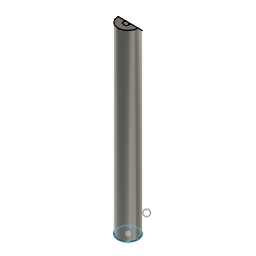
solarpanel (Autodesk Fusion 360 archive; units mm, degrees)
design "Stepper_Motor_Pole_Solar_Panel"
part number: 2025-08-02-13-12-08-452
Autodesk Fusion 360 part; units mm, degrees
sketch "Skizze1" plane through (0, 0, 0) normal (0, 0, 1) x (1, 0, 0)
  point P0 (-5.2, 16.4)
sketch "Skizze2" plane through (0, 0, 0) normal (0, 0, 1) x (1, 0, 0)
  circle A0 centre (0, 0) radius 6
extrude "Extrusion2" add sketch "Skizze2" along normal blind 110
sketch "Skizze3" plane through (0, 0, 0) normal (0, 0, 1) x (1, 0, 0)
  line L0 (-1.5, -2) -> (-1.5, 2)
  line L1 (1.5, -2) -> (1.5, 2)
  arc A0 (-1.5, -2) -> (1.5, -2) centre (0, 0) ccw
  arc A1 (1.5, 2) -> (-1.5, 2) centre (0, 0) ccw
  dimension "d15" = 5
  constraint coincident A0.centre A1.centre
  constraint coincident L1.end A0
  constraint concentric A0 A1
  measures "d15" diameter of A0
extrude "Extrusion3" cut sketch "Skizze3" along normal blind 20
pattern_linear "R-Anordnung1" count 2 spacing 98 along (0, 0, 1) of "Extrusion3"
ref_plane "Arbeitsebene1" through (-6, 0, 108.0306) normal (-1, 0, 0) x (0, 1, 0)
sketch "Skizze5" plane through (-6, 0, 0) normal (-1, 0, 0) x (0, -1, 0)
  line L0 (0, 110) -> (-6.178, 103.822)
  line L1 (-6.178, 103.822) -> (-6.178, 110)
  line L2 (-6.178, 110) -> (0, 110)
  constraint perpendicular L1 L2
extrude "Extrusion4" cut sketch "Skizze5" against normal blind 100

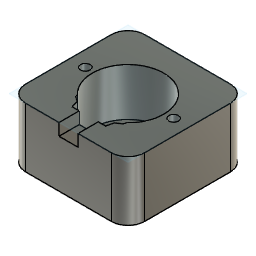
design "Stepper_Motor_Solar_Panel"
part number: 2025-07-29-17-04-06-357
Autodesk Fusion 360 part; units mm, degrees
sketch "Skizze1" plane through (0, 0, 0) normal (0, 0, 1) x (1, 0, 0)
  line L0 (0, 0) -> (50, 0)
  line L1 (50, 0) -> (50, 50)
  line L2 (50, 50) -> (0, 50)
  line L3 (0, 50) -> (0, 0)
  dimension "d1" = 50
  dimension "d2" = 50
  constraint horizontal L0
  constraint vertical L1
  constraint horizontal L2
  constraint vertical L3
  constraint coincident L0.start L3.end
  measures "d1" distance of L0.start L0.end
  measures "d2" distance of L0.start L2.end
extrude "Extrusion1" add sketch "Skizze1" along normal blind 25
sketch "Skizze4" plane through (0, 0, 25) normal (0, 0, 1) x (-1, 0, 0)
  line L0 (0, -50) -> (0, 0)
  line L1 (0, 0) -> (-50, 0)
  line L2 (-50, 0) -> (-50, -50)
  line L3 (-50, -50) -> (0, -50)
sketch "Skizze5" plane through (0, 0, 25) normal (0, 0, 1) x (-1, 0, 0)
  line L0 (0, 0) -> (-50, 0)
  line L1 (-28.9998, -8.5) -> (-28.9998, 0)
  line L2 (-32.7998, -11.4915) -> (-35, -13)
  line L3 (-35, -13) -> (-36, -18)
  line L4 (-24.9998, -16.7741) -> (-24.9998, -8.5)
  line L5 (-24.9998, -16.7741) -> (-24.9998, -8.5)
  line L6 (-17.1998, -11.4915) -> (-14.9997, -13)
  line L7 (-14.9997, -13) -> (-13.9997, -18)
  line L8 (-28.9998, 0) -> (-20.9998, 0)
  line L9 (-20.9998, 0) -> (-20.9998, -8.5)
  line L10 (-24.9998, -8.5) -> (-17.9498, -8.5)
  line L11 (-32.0498, -8.5) -> (-24.9998, -8.5)
  line L12 (-17.1998, -11.4915) -> (-17.9498, -8.5)
  line L13 (-32.7998, -11.4915) -> (-32.0498, -8.5)
  line L14 (-13.9997, -18) -> (-36, -18)
  dimension "d43" = 8
  dimension "d46" = 7.05
  dimension "d47" = 7.05
  dimension "d48" = 2.9915
  dimension "d49" = 2.9915
  constraint coincident L0 L1.end
  constraint perpendicular L0 L1
  constraint symmetric L2.start L4 L6.start
  constraint symmetric L3.end L4 L7.end
  constraint symmetric L5.start L4 L4.start
  constraint symmetric L5.end L4 L10.start
  constraint symmetric L2.end L4 L6.end
  constraint perpendicular L1 L8
  constraint perpendicular L9 L10
  constraint horizontal L14
  measures "d43" distance of L1.end L8.end
  measures "d46" distance of L4.end L10.end
  measures "d47" distance of L4.end L11.start
  measures "d48" vertical distance of L6.start L10.end
  measures "d49" vertical distance of L2.start L11.start
extrude "Extrusion3" cut sketch "Skizze5" against normal blind 20 contours L2 L3 L6 L7 L10 L11 L12 L13 L14
sketch "Skizze6" plane through (0, 0, 25) normal (0, 0, 1) x (-1, 0, 0)
  circle A0 centre (-25, -25) radius 15
  dimension "d36" = 30
  measures "d36" diameter of A0
extrude "Extrusion4" cut sketch "Skizze6" against normal blind 20
sketch "Skizze7" plane through (0, 0, 25) normal (0, 0, 1) x (-1, 0, 0)
  circle A0 centre (-6.431, -25.6214) radius 2
  line L0 (-25, 0) -> (-25, -50)
  circle A1 centre (-43.569, -25.6214) radius 2
  dimension "d17" = 4
  dimension "d39" = 50
  constraint vertical L0
  constraint symmetric A0 L0 A1
  measures "d17" diameter of A0
  measures "d39" distance of L0.start L0.end
extrude "Extrusion5" cut sketch "Skizze7" against normal blind 20
sketch "Skizze10" plane through (0, 0, 25) normal (0, 0, 1) x (-1, 0, 0)
fillet "Abrundung1" radius 7 4 edges at (50, 50, 12.5) (50, 0, 12.5) (0, 50, 12.5) (0, 0, 12.5)
extrude "Extrusion6" cut sketch "Skizze5" against normal blind 4 contours L0 L1 L8 L9 L10 L11
extrude "Extrusion7" cut sketch "Skizze5" against normal blind 5 contours L0 L1 L8 L9 L10 L11
sketch "Skizze11" plane through (0, 0, 25) normal (0, 0, 1) x (-1, 0, 0)

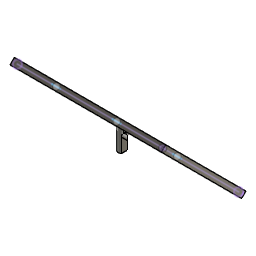
design "Top_Solar_Panel"
part number: 2025-08-20-09-59-22-880
Autodesk Fusion 360 part; units mm, degrees
sketch "Skizze1" plane through (0, 0, 0) normal (0, 0, 1) x (1, 0, 0)
  line L0 (1.5, -2) -> (1.5, 2)
  line L1 (-1.5, -2) -> (-1.5, 2)
  arc A0 (-1.5, -2) -> (1.5, -2) centre (0, 0) ccw
  arc A1 (1.5, 2) -> (-1.5, 2) centre (0, 0) ccw
  dimension "d1" = 5
  constraint coincident A0.centre A1.centre
  constraint coincident L0.end A0
  constraint vertical L1
  constraint concentric A0 A1
  measures "d1" diameter of A0
extrude "Extrusion1" add sketch "Skizze1" along normal blind 12
ref_plane "Arbeitsebene1" through (0, 0, 0) normal (1, 0, 0) x (0, 1, 0)
sketch "Skizze3" plane through (0, 0, 12) normal (0, 0, 1) x (-1, 0, 0)
  line L0 (1.5, -2) -> (1.5, 2)
  arc A0 (1.5, 2) -> (-1.5, 2) centre (0, 0) ccw
  line L1 (-1.5, 2) -> (-1.5, -2)
  circle A1 centre (0, 0) radius 6
  arc A2 (-1.5, -2) -> (1.5, -2) centre (0, 0) ccw
  constraint concentric A0 A1
ref_plane "Arbeitsebene2" through (0, 3, 8.9997) normal (0, -0.707147, -0.707067) x (0, 0.707067, -0.707147)
sketch "Skizze5" plane through (0, 6, 5.9993) normal (0, -0.707147, -0.707067) x (0, 0.707067, -0.707147)
  line L0 (-42.5, 50) -> (32.5, 50)
  line L1 (32.5, 50) -> (32.5, -50)
  line L2 (32.5, -50) -> (-42.5, -50)
  line L3 (-42.5, -50) -> (-42.5, 50)
  line L4 (-42.5, 50) -> (32.5, -50) construction
  line L5 (32.5, 50) -> (-42.5, -50) construction
  point P0 (-5, 0)
  dimension "d45" = 100
  dimension "d46" = 75
  constraint horizontal L0
  constraint perpendicular L0 L1
  constraint parallel L0 L2
  constraint parallel L1 L3
  constraint coincident L4 P0
  constraint coincident L5 P0
  measures "d45" distance of L0.start L2.end
  measures "d46" distance of L0.start L0.end
extrude "Extrusion4" add sketch "Skizze5" against normal blind 4
shell "Schale1" thickness 2 removed faces 1 at (-16.6667, 14.1316, 3.524)
fillet "Abrundung1" radius 3.25 2 edges at (1.5, 1, 10.9999) (-1.5, 1, 10.9999)
fillet "Abrundung2" radius 1.25 1 edges at (0, 2.5, 9.4997)
extrude "Extrusion5" add 1 faces at (0.0599, -0.8312, 12) along direction (0, 0, 1) blind 2.5
sketch "Skizze6" plane through (0, 7.4143, 7.4135) normal (0, 0.707147, 0.707067) x (-1, 0, 0)
  line L0 (48, -30.5) -> (48, 40.5)
  line L1 (48, 40.5) -> (-48, 40.5)
  line L2 (-48, 40.5) -> (-48, -30.5)
  line L3 (-48, -30.5) -> (48, -30.5)
  dimension "d25" = 96
  dimension "d26" = 71
  measures "d25" distance of L0.end L1.end
  measures "d26" distance of L1.end L2.end
sketch "Skizze7" plane through (0, 7.4143, 7.4135) normal (0, 0.707147, 0.707067) x (-1, 0, 0)
  line L0 (48, 40.5) -> (-48, 40.5)
  line L1 (-48, 40.5) -> (-48, -30.5)
  circle A0 centre (0.1555, 15.2617) radius 2.5
  circle A1 centre (-39.8445, 15.2617) radius 2.5
  circle A2 centre (40.1555, 15.2617) radius 2.5
  dimension "d28" = 96
  dimension "d29" = 71
  dimension "d30" = 5
  dimension "d49" = 40
  dimension "d50" = 0
  measures "d28" distance of L0.start L0.end
  measures "d29" distance of L0.end L1.end
  measures "d30" diameter of A0
extrude "Extrusion9" cut sketch "Skizze7" against normal blind 10 contours A0
extrude "Extrusion10" cut sketch "Skizze7" against normal blind 30 contours A1 | A2
